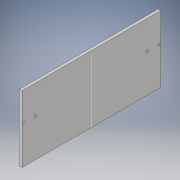
# Autodesk Inventor part: SuspensionDrivePlate
Saved by Autodesk Inventor 2017 (Build 210142000, 142)
## iProperties
Created: 2018-05-09
Part Number: SuspensionDrivePlate
Material: Generic
Document SubType Name: Modeling
Designer: User
Density: 1 g/cm^3
Appearance: Default
Author: User
Autodesk Inventor part; units mm, degrees
ref_plane "YZ Plane" through (0, 0, 0) normal (1, 0, 0) x (0, 1, 0)
ref_plane "XZ Plane" through (0, 0, 0) normal (0, 1, 0) x (-1, 0, 0)
ref_plane "XY Plane" through (0, 0, 0) normal (0, 0, 1) x (1, 0, 0)
sketch "Sketch1" plane through (0, 0, 0) normal (1, 0, 0) x (0, 1, 0)
  line L0 (0, 0) -> (111.125, 0)
  line L1 (111.125, 0) -> (111.125, -231.775)
  line L2 (111.125, -231.775) -> (0, -231.775)
  line L3 (0, -231.775) -> (0, 0)
  dimension "d0" = 111.125
  dimension "d1" = 231.775
  constraints: 8 end point, 2 parallel, 1 horizontal, 1 perpendicular
  measures "d0" distance of L1.end L2.end
  measures "d1" distance of L0.end L1.end
extrude "Extrusion1" add sketch "Sketch1" along normal blind 4.7625
sketch "Sketch2" plane through (4.7625, 0, 0) normal (1, 0, 0) x (0, 0, -1)
  line L0 (0, 111.125) -> (0, 0) projected
  line L1 (0, 0) -> (231.775, 0) projected
  line L2 (231.775, 0) -> (231.775, 111.125) projected
  line L3 (231.775, 111.125) -> (0, 111.125) projected
  point P0 (3.175, 63.5)
  point P1 (22.225, 63.5)
  point P2 (209.55, 63.5)
  point P3 (228.6, 63.5)
  dimension "d4" = 63.5
  dimension "d5" = 63.5
  dimension "d6" = 63.5
  dimension "d7" = 63.5
  dimension "d8" = 3.175
  dimension "d9" = 19.05
  dimension "d10" = 19.05
  dimension "d11" = 3.175
  measures "d4" distance from line of L1 point (3.175, 63.5)
  measures "d5" distance from line of L1 point (22.225, 63.5)
  measures "d6" distance from line of L1 point (209.55, 63.5)
  measures "d7" distance from line of L1 point (228.6, 63.5)
  measures "d8" distance from line of point (3.175, 63.5) L0
  measures "d9" distance of point (22.225, 63.5) point (3.175, 63.5)
  measures "d10" distance of point (228.6, 63.5) point (209.55, 63.5)
  measures "d11" distance from line of L2 point (228.6, 63.5)
hole "Hole1" at (4.7625, 63.5, -3.175) at (4.7625, 63.5, -22.225) at (4.7625, 63.5, -209.55) at (4.7625, 63.5, -228.6) direction (-1, 0, 0) diameter 3.683 depth 25.4 tip angle 118
ref_plane "Work Plane1" through (0, 0, -115.8875) normal (0, 0, 1) x (1, 0, 0)
equation "\"d5\" = d4"
equation "\"d6\" = d4"
equation "\"d7\" = d4"
equation "\"d10\" = d9"
equation "\"d11\" = d8"
body "Solid1"
